Autodesk Fusion 360 part; units mm, degrees
note: some values were not read from the file. Set by a fixed rule: which face or edge a step refers to.
(part 3 of 3)
  arc A214 (87.3364, -31.9587) -> (92.3976, -10.5682) centre (0, 0) ccw
  arc A215 (35.1534, 80.8919) -> (37.1429, 72.8829) centre (42.7998, 78.5398) ccw
  line L68 (37.1429, 72.8829) -> (43.1865, 66.8393)
  arc A216 (43.1865, 62.5966) -> (43.1865, 66.8393) centre (41.0652, 64.7179) ccw
  line L69 (43.1865, 62.5966) -> (39.5745, 58.9846)
  arc A217 (32.9007, 58.6276) -> (39.5745, 58.9846) centre (36.039, 62.5201) ccw
  arc A218 (32.9007, 58.6276) -> (29.5638, 58.4491) centre (31.3316, 56.6814) ccw
  line L70 (29.5638, 58.4491) -> (26.7937, 55.679)
  arc A219 (24.5671, 55.2656) -> (26.7937, 55.679) centre (25.3795, 57.0932) ccw
  arc A220 (24.5671, 55.2656) -> (9.6799, 59.7003) centre (0, 0) ccw
  arc A221 (8, 61.6746) -> (9.6799, 59.7003) centre (10, 61.6746) ccw
  line L71 (8, 61.6746) -> (8, 87.43)
  arc A222 (10.2273, 89.417) -> (8, 87.43) centre (10, 87.43) ccw
  arc A223 (33.9973, 83.3318) -> (10.2273, 89.417) centre (0, 0) ccw
  arc A224 (35.1534, 80.8919) -> (33.9973, 83.3318) centre (33.2418, 81.48) ccw
move_body "移動1" bodies 1 to x (-1, 0, 0) y (0, 1, 0) z (0, 0, -1) at (0, 0, 0)
move_body "移動2" bodies 1 to x (-1, 0, 0) y (0, 1, 0) z (0, 0, -1) at (0, 0, 0)
